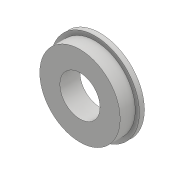
# Autodesk Inventor part: ベアリング12x18
Saved by Autodesk Inventor 2020.3 (Build 243373000, 373)
## iProperties
Part Number: ベアリング12x18
Material: 一般
Document SubType Name: Modeling
Designer: highs
Density: 1 g/cm^3
Appearance: 既定
Author: highs
Autodesk Inventor part; units mm, degrees
ref_plane "YZ Plane" through (0, 0, 0) normal (1, 0, 0) x (0, 1, 0)
ref_plane "XZ Plane" through (0, 0, 0) normal (0, 1, 0) x (-1, 0, 0)
ref_plane "XY Plane" through (0, 0, 0) normal (0, 0, 1) x (1, 0, 0)
sketch "スケッチ1" plane through (0, 0, 0) normal (0, 0, 1) x (1, 0, 0)
  line L0 (0, 0) -> (6, 0) construction
  line L1 (6, 0) -> (6, 6)
  line L2 (6, 6) -> (13.25, 6)
  line L3 (13.25, 6) -> (13.25, 4.5)
  line L4 (13.25, 4.5) -> (12, 4.5)
  line L5 (12, 4.5) -> (12, 0)
  line L6 (12, 0) -> (6, 0)
  line L7 (0, 0) -> (0, 6) construction
  line L8 (0, 6) -> (6, 6) construction
  dimension "d0" = 6
  dimension "d1" = 12
  dimension "d2" = 1.5
  dimension "d3" = 13.25
  dimension "d4" = 6
  constraints: 18 end point, 7 perpendicular, 1 horizontal, 1 point on line, 1 vertical
  measures "d0" distance from line of L0.start L1
  measures "d1" distance from line of L0.start L5
  measures "d2" distance of L2.end L3.end
  measures "d3" distance from line of L0.start L3
  measures "d4" distance between parallel lines of L6 L2
revolve "回転1" add sketch "スケッチ1" angle 360 about axis through (0, 0, 0) along (0, 1, 0)
